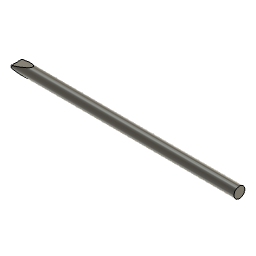
screwdriver_assy v1 (Autodesk Fusion 360 archive; units mm, degrees)
design "screwdriver schaft"
Autodesk Fusion 360 part; units mm, degrees
sketch "Sketch1" plane through (0, 0, 0) normal (0, 1, 0) x (1, 0, 0)
  line L0 (0, 0) -> (95, 0)
  line L1 (95, 0) -> (95, -2.3)
  line L2 (0, 0) -> (0, -2.3)
  line L3 (0, -2.3) -> (95, -2.3)
  dimension "d1" = 95
  dimension "d6" = 2.3
  constraint horizontal L0
  constraint vertical L1
  constraint coincident L0.start L2.start
  constraint perpendicular L0 L2
  constraint perpendicular L1 L3
  measures "d1" distance of L0.start L0.end
  measures "d6" distance of L0.start L2.end
revolve "Revolve1" add sketch "Sketch1" angle 360 about axis through (0, 0, 0) along (1, 0, 0)
sketch "Sketch3" plane through (0, 0, 0) normal (0, 1, 0) x (1, 0, 0)
  line L0 (0, 0) -> (95, 0) construction
  line L1 (95, 0) -> (0, 0) construction
  line L2 (0, 0) -> (0, -2.3) construction
  line L3 (0, -2.3) -> (0, -0.5)
  line L4 (0, -2.3) -> (7, -2.3)
  line L5 (7, -2.3) -> (0, -0.5)
  line L6 (0, 2.3) -> (0, 0.5)
  line L7 (7, 2.3) -> (0, 0.5)
  line L8 (0, 2.3) -> (7, 2.3)
  dimension "d20" = 2.3
  dimension "d21" = 1.8
  dimension "d22" = 7
  constraint coincident L0.start L1.end
  constraint horizontal L0
  constraint perpendicular L0 L2
  constraint parallel L2 L3
  constraint perpendicular L3 L4
  constraint symmetric L1 L2.end L6.start
  constraint symmetric L1 L3.end L6.end
  constraint symmetric L1 L4.end L7.start
  measures "d20" distance of L0.start L2.end
  measures "d21" distance of L2.end L3.end
  measures "d22" distance of L2.end L4.end
extrude "Extrude1" cut sketch "Sketch3" along normal mid plane 10
